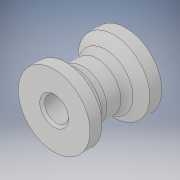
# Autodesk Inventor part: Qatest-Stock Transfer
Saved by Autodesk Inventor 2019 (Build 230136000, 136)
## iProperties
Created: 2016-09-01
Part Number: Qatest-Stock Transfer
Material: Generic
Document SubType Name: Modeling
Designer: Awhatmough
Density: 1 g/cm^3
Appearance: Default
Author: Awhatmough
Autodesk Inventor part; units mm, degrees
ref_plane "YZ Plane" through (0, 0, 0) normal (1, 0, 0) x (0, 1, 0)
ref_plane "XZ Plane" through (0, 0, 0) normal (0, 1, 0) x (-1, 0, 0)
ref_plane "XY Plane" through (0, 0, 0) normal (0, 0, 1) x (1, 0, 0)
sketch "Sketch1" plane through (0, 0, 0) normal (1, 0, 0) x (0, 1, 0)
  line L0 (0, 0) -> (0, -19.05)
  line L1 (0, -19.05) -> (9.525, -19.05)
  line L2 (9.525, -19.05) -> (9.525, -15.875)
  line L3 (9.525, -15.875) -> (6.35, -12.7)
  line L4 (6.35, -12.7) -> (6.35, -6.35)
  line L5 (6.35, -6.35) -> (9.525, -3.175)
  line L6 (9.525, -3.175) -> (9.525, 0)
  line L7 (9.525, 0) -> (0, 0)
  line L8 (6.35, -9.525) -> (12.7302, -9.525) construction
  dimension "d1" = 9.525
  dimension "d2" = 135
  dimension "d3" = 19.05
  dimension "d4" = 6.35
  dimension "d5" = 3.175
  constraints: 18 end point, 4 perpendicular, 1 collinear, 1 horizontal, 1 midpoint, 1 parallel, 1 point on line, 1 vertical
  measures "d1" distance between parallel lines of L6 L0
  measures "d2" angle of L6 L5
  measures "d3" distance of L0.start L0.end
  measures "d4" distance of L3.end L4.end
  measures "d5" horizontal distance of L4.end L5.end
revolve "Revolution1" add sketch "Sketch1" angle 360 about axis through (0, 0, 0) along (0, 0, -1)
sketch "Sketch2" plane through (0, 0, -19.05) normal (0, 0, -1) x (-1, 0, 0)
  circle A0 centre (0, 0) radius 3.175
  dimension "d7" = 6.35
  constraints: 1 centre point, 1 coincident
  measures "d7" diameter of A0
extrude "Extrusion1" cut sketch "Sketch2" against normal through all
chamfer "Chamfer1" distance 0.635 angle 45 2 edges at (3.175, 0, -19.05) (3.175, 0, 0)
fillet "Fillet1" radius 3.175 2 edges at (0, -6.35, -6.35) (0, -6.35, -12.7)
body "Solid1"
